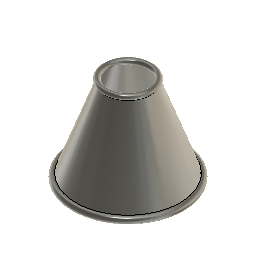
Lamp v1 (Autodesk Fusion 360 design; units mm, degrees)
Autodesk Fusion 360 part; units mm, degrees
sketch "Sketch1" plane through (0, 0, 0) normal (0, 1, 0) x (1, 0, 0)
  line L0 (8.6695, -31.203) -> (19.8347, -0.5268)
  line L1 (19.4228, -0.6284) -> (8.2576, -31.3046)
  circle A0 centre (8.2865, -32.1436) radius 1.0155
  circle A1 centre (19.8999, -0.3139) radius 1.25
  dimension "d5" = 2.5
  constraint coincident L0.start A0
  measures "d5" diameter of A1
revolve "Revolve1" add sketch "Sketch1" angle 360 about axis through (0, 0, 1.75) along (0, 0, 1)
